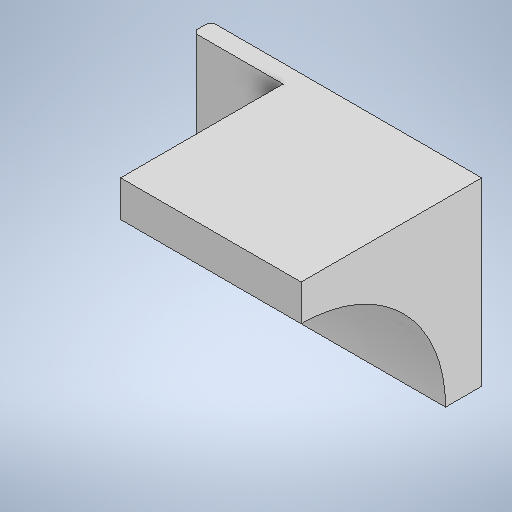
# Autodesk Inventor part: flat_surface_1
Saved by Autodesk Inventor 2025 (Build 290162010, 162A)
## iProperties
Created: 2025-06-15
Part Number: flat_surface_1
Material: 일반
Document SubType Name: Modeling
Designer: USER
Density: 1 g/cm^3
Appearance: 기본값
Author: USER
Autodesk Inventor part; units mm, degrees
ref_plane "YZ Plane" through (0, 0, 0) normal (1, 0, 0) x (0, 1, 0)
ref_plane "XZ Plane" through (0, 0, 0) normal (0, 1, 0) x (-1, 0, 0)
sketch "스케치1" plane through (0, 0, 0) normal (0, 0, 1) x (1, 0, 0)
  line L0 (-0.15, 0) -> (0.9, 0) construction
  line L1 (0, -0.7) -> (0, 0.7) construction
  line L2 (0.25, -0.5) -> (0.75, -0.5)
  line L3 (0.75, -0.5) -> (0.75, 0.5)
  line L4 (0.75, 0.5) -> (0.25, 0.5)
  line L5 (0.25, 0.5) -> (0.25, -0.5)
  point P0 (0, 0)
  point P1 (0.5, -0.5)
  dimension "d7" = 0.5
  dimension "d8" = 1
  dimension "d9" = 0.25
  constraints: 8 end point, 2 parallel, 1 horizontal, 1 midpoint, 1 perpendicular, 1 other
  measures "d7" distance between parallel lines of L5 L3
  measures "d8" distance between parallel lines of L2 L4
  measures "d9" distance between parallel lines of L1 L5
extrude "돌출1" add sketch "스케치1" along normal blind 0.1
sketch "스케치3" plane through (0.25, 0.5, 0) normal (0, 1, 0) x (1, 0, 0)
  line L0 (-0.25, 0.7571) -> (-0.25, -0.2929) construction
  line L1 (-0.4, 0) -> (0.65, 0) construction
  line L2 (0.5, 0) -> (0, 0) projected
  line L3 (0, 0) -> (0, -0.1) projected
  line L4 (0.5, -0.1) -> (0, -0.1) projected
  line L5 (0.5, 0) -> (0.5, -0.1) projected
  arc A0 (0, -0.1) -> (0.5, -0.1) centre (0.25, 0.6071) ccw
  line L6 (0.25, -0.1) -> (0.25, 0.4799) construction
  point P0 (-0.25, 0)
  dimension "d10" = 0.75
  constraints: 2 end point, 2 point on circle, 1 centre point, 1 midpoint, 1 point on line, 1 vertical
  measures "d10" radius of A0
sketch "스케치5" plane through (0, 0, 0.1) normal (0, 0, 1) x (1, 0, 0)
  line L0 (0.75, -0.5) -> (0.75, 0.5) projected
  line L1 (0.75, 0.5) -> (0.25, 0.5) projected
  line L2 (0.25, 0.5) -> (0.25, -0.5) projected
  line L3 (0.25, -0.5) -> (0.75, -0.5) projected
  line L4 (-0.15, 0) -> (0.9, 0) construction
  line L5 (0, -0.7) -> (0, 0.7) construction
  line L6 (-0.15, 0) -> (0.9, 0) construction
  line L7 (0, 0.7) -> (0, -0.7) construction
  line L8 (0.75, 0.4) -> (0.25, 0.4)
  line L9 (0.75, -0.4) -> (0.25, -0.4)
  point P0 (0, 0)
  dimension "d18" = 1
  dimension "d19" = 0.4
  constraints: 4 end point, 2 point on line, 2 symmetric about line, 1 perpendicular
  measures "d18" distance between parallel lines of L1 L3
  measures "d19" distance between parallel lines of L4 L8
sketch "스케치6" plane through (0.75, -0.5, 0) normal (1, 0, 0) x (0, 0, -1)
  line L0 (0, 0) -> (0, 1) projected
  line L1 (0, 1) -> (-0.1, 1) projected
  line L2 (-0.1, 0) -> (-0.1, 1) projected
  line L3 (0, 0) -> (-0.1, 0) projected
  line L4 (0, 0.5) -> (-0.1, 0.5) construction
  line L5 (0, 0.92) -> (-0.1, 0.92)
  arc A0 (-0.1, 0.92) -> (-0.02, 1) centre (-0.1, 1) ccw
  arc A1 (-0.02, 0) -> (-0.1, 0.08) centre (-0.1, 0) ccw
  point P0 (-0.05, 0.5)
  point P1 (-0.05, 0.92)
  point P2 (-0.02, 0)
  point P3 (-0.1, 0.08)
  dimension "d20" = 0.42
  constraints: 4 end point, 4 point on circle, 3 midpoint, 3 point on line, 3 symmetric about line, 2 centre point, 1 coincident, 1 perpendicular, 1 other
  measures "d20" distance of point (-0.05, 0.5) point (-0.05, 0.92)
extrude "돌출5" cut sketch "스케치6" against normal up to surface (0.5 mm away) contours L3 L2 A1 | L2 L1 A0
sketch "스케치7" plane through (0.75, -0.5, 0) normal (1, 0, 0) x (0, 0, -1)
  arc A0 (-0.1, 0.92) -> (-0.02, 1) centre (-0.1, 1) ccw projected
  line L0 (-0.1, 0.08) -> (-0.1, 0.92) projected
  arc A1 (-0.02, 0) -> (-0.1, 0.08) centre (-0.1, 0) ccw projected
  line L1 (0, 0) -> (-0.02, 0) projected
  line L2 (0, 0) -> (0, 1) projected
  line L3 (0, 1) -> (-0.02, 1) projected
  line L4 (0, 0.5) -> (-0.2526, 0.5) construction
  line L5 (-0.2526, 0.5) -> (-0.2526, 0.9) construction
  line L6 (-0.2526, 0.9) -> (-0.1, 0.9) construction
  line L7 (-0.2526, 0.1) -> (-0.1, 0.1) construction
  dimension "d23" = 0.4
  constraints: 8 end point, 2 symmetric about line, 1 horizontal, 1 perpendicular, 1 point on line, 1 vertical
  measures "d23" distance of L4.end L5.end
ref_plane "작업 평면1" through (0.25, -0.4, 0) normal (0, -1, 0) x (1, 0, 0)
sketch "스케치8" plane through (0.25, -0.4, 0) normal (0, -1, 0) x (1, 0, 0)
  line L0 (0, 0.02) -> (0, 0.1) projected
  line L1 (0.5, 0.02) -> (0, 0.02) projected
  line L2 (0.5, 0.1) -> (0.5, 0.02) projected
  line L3 (0, 0.1) -> (0.5, 0.1) projected
  line L4 (0.5, 0.02) -> (0, 0.02) projected
  line L5 (0, 0) -> (0, 0.02) projected
  line L6 (0, 0) -> (0.5, 0) projected
  line L7 (0.5, 0) -> (0.5, 0.02) projected
  point P0 (-0.25, 0)
  point P1 (0.5, 0.02)
  point P2 (0, 0.02)
extrude "돌출6" cut sketch "스케치8" against normal blind 10
sketch "스케치9" plane through (0.25, -0.4, 0) normal (0, 1, 0) x (1, 0, 0)
  line L0 (0.5, 0) -> (0.5, -0.1) projected
  line L1 (0, 0) -> (0.5, 0) projected
  line L2 (0, -0.1) -> (0, 0) projected
  line L3 (0.5, -0.1) -> (0, -0.1) projected
  line L4 (0, 0) -> (0.5, 0) construction
  line L5 (0.2, 0) -> (0.2, -0.1) construction
  line L6 (0.2, -0.1) -> (0.2, -0.0922)
  line L7 (0.2, -0.01) -> (0.15, -0.01)
  line L8 (0.15, -0.01) -> (0.15, 0)
  line L9 (0.4, 0) -> (0.4, -0.1) construction
  line L10 (0.5, -0.1) -> (0, -0.1) construction
  line L11 (0.4, -0.01) -> (0.35, -0.01)
  line L12 (0.35, -0.01) -> (0.35, 0)
  line L13 (0.4, -0.01) -> (0.4, -0.1)
  line L14 (0.2, -0.01) -> (0.2, -0.1)
  point P0 (-0.25, 0)
  point P1 (0, -0.05)
  dimension "d27" = 0.2
  dimension "d28" = 0.01
  dimension "d29" = 0.2
  dimension "d30" = 0.05
  dimension "d31" = 0.05
  constraints: 18 end point, 9 point on line, 6 perpendicular, 1 collinear, 1 horizontal, 1 midpoint, 1 parallel
  measures "d27" distance from line of point (0, -0.05) L5
  measures "d28" distance between parallel lines of L1 L7
  measures "d29" distance between parallel lines of L9 L5
  measures "d30" distance between parallel lines of L5 L8
  measures "d31" distance between parallel lines of L9 L12
extrude "돌출7" cut sketch "스케치9" against normal blind 10 contours L12 L11 L13 L3 L6 L14 L7 L8 L1 | L8 L7 L14 L6 L3 L2 L1
chamfer "모따기1" distance 0.002 angle 45 2 edges at (0.6, -0.45, 0) (0.6, -0.45, 0.01)
sketch "스케치10" plane through (0.65, -0.4, 0.01) normal (-1, 0, 0) x (0, 0, 1)
  line L0 (0.01, -0.1) -> (0, -0.1) projected
  arc A0 (0.09, -0.02) -> (0.01, -0.1) centre (0.09, -0.1) ccw projected
  line L1 (0.09, 0) -> (0.09, -0.02) projected
  line L2 (0, 0) -> (0.09, 0) projected
  line L3 (0, 0) -> (0, -0.1) projected
  line L4 (0, -0.02) -> (0.02, -0.02) construction
  line L5 (0.02, -0.02) -> (0.02, 0) construction
  circle A1 centre (0.02, -0.02) radius 0.0015
  point P0 (-0.01, 0.4)
  dimension "d37" = 0.02
  dimension "d38" = 0.02
  dimension "d39" = 0.003
  constraints: 4 end point, 2 point on line, 1 centre point, 1 coincident, 1 horizontal, 1 perpendicular
  measures "d37" distance between parallel lines of L3 L5
  measures "d38" distance between parallel lines of L2 L4
  measures "d39" diameter of A1
extrude "돌출8" cut sketch "스케치10" against normal blind 0.003 contours A1
